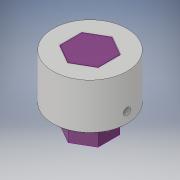
# Autodesk Inventor part: Wheel
Saved by Autodesk Inventor 2019.2 (Build 232265000, 265)
## iProperties
Created: 2019-05-20
Part Number: Wheel
Material: Generic
Document SubType Name: Modeling
Designer: Johansson
Density: 1 g/cm^3
Appearance: Default
Author: Johansson
## iProperties of the stored document Wheel_3DPrint.ipt
Created: 2019-05-23
Part Number: Wheel_3DPrint
Material: Generic
Document SubType Name: Modeling
Designer: Johansson
Density: 1 g/cm^3
Appearance: Default
Author: Johansson
Autodesk Inventor part; units mm, degrees
ref_plane "YZ Plane" through (0, 0, 0) normal (1, 0, 0) x (0, 1, 0)
ref_plane "XZ Plane" through (0, 0, 0) normal (0, 1, 0) x (-1, 0, 0)
ref_plane "XY Plane" through (0, 0, 0) normal (0, 0, 1) x (1, 0, 0)
sketch "Sketch1" plane through (0, 0, 0) normal (0, 1, 0) x (-1, 0, 0)
  circle A0 centre (0, 0) radius 4.1
  line L0 (8.2, 4.7343) -> (8.2, -4.7343)
  line L1 (8.2, -4.7343) -> (0, -9.4685)
  line L2 (0, -9.4685) -> (-8.2, -4.7343)
  line L3 (-8.2, -4.7343) -> (-8.2, 4.7343)
  line L4 (-8.2, 4.7343) -> (0, 9.4685)
  line L5 (0, 9.4685) -> (8.2, 4.7343)
  dimension "d1" = 8.2
  dimension "d5" = 8.2
  constraints: 12 end point, 2 coincident, 1 centre point, 1 vertical, 13 other
  measures "d1" diameter of A0
  measures "d5" distance from line of point (0, 0) L0
extrude "Extrusion1" add sketch "Sketch1" along normal blind 20
sketch "Sketch2" plane through (-8.2, 0, -4.7343) normal (-1, 0, 0) x (0, 0, 1)
  circle A0 centre (4.7343, 5) radius 1.5
  line L0 (9.4685, 0) -> (0, 0) projected
  line L1 (4.7343, -4) -> (4.7343, 24) projected
  point P0 (4.7343, 0)
  dimension "d6" = 3
  dimension "d7" = 5
  constraints: 1 centre point, 1 point on line
  measures "d6" diameter of A0
  measures "d7" distance from line of A0.centre L0
extrude "Extrusion2" cut sketch "Sketch2" against normal through all
ref_plane "Work Plane1" through (0, 10, 0) normal (0, -1, 0) x (1, 0, 0)
mirror "Mirror1" about plane through (0, 10, 0) normal (0, -1, 0) of "Extrusion2"
sketch "Sketch3" plane through (0, 20, 0) normal (0, 1, 0) x (1, 0, 0)
  circle A0 centre (0, 0) radius 4.1 projected
  line L0 (-8.2, 4.7343) -> (-8.2, -4.7343) projected
  line L1 (-8.2, -4.7343) -> (0, -9.4685) projected
  line L2 (0, -9.4685) -> (8.2, -4.7343) projected
  line L3 (8.2, -4.7343) -> (8.2, 4.7343) projected
  line L4 (8.2, 4.7343) -> (0, 9.4685) projected
  line L5 (0, 9.4685) -> (-8.2, 4.7343) projected
  circle A1 centre (0, 0) radius 16
  dimension "d10" = 32
  constraints: 1 centre point, 1 coincident
  measures "d10" diameter of A1
extrude "Extrusion3" add sketch "Sketch3" along normal blind 10 and the other way blind 10 separate body contours A1
thicken "Thicken1" operation add thickness 0.2 both sides no extend neighbours yes toward (0.5, 0, 0.8660254) bodies 2 faces at (2.7333, 23.3333, 7.8905) (2.7333, 16.6667, 7.8905) (-5.4667, 23.3333, 6.3124) (-5.4667, 16.6667, 6.3124) (-8.2, 23.3333, -1.5781) (-8.2, 16.6667, -1.5781) (-2.7333, 26.6667, -7.8905) (-2.7333, 13.3333, -7.8905) (5.4667, 23.3333, -6.3124) (5.4667, 16.6667, -6.3124) (8.2, 23.3333, 1.5781) (8.2, 16.6667, 1.5781)
ref_plane "Work Plane2" through (-16, 20, 0) normal (-1, 0, 0) x (0, -1, 0)
sketch "Sketch4" plane through (-16, 20, 0) normal (-1, 0, 0) x (0, -1, 0)
  circle A0 centre (5, 0) radius 1.5 projected
  point P0 (20, 0)
extrude "Extrusion4" cut sketch "Sketch4" against normal through all bodies 2
sketch "Sketch5" plane through (-8.2, 20, 4.7343) normal (0, 1, 0) x (1, 0, 0)
  point P0 (8.2, 4.7343)
sketch "Sketch6" plane through (0, 20, 0) normal (0, 1, 0) x (1, 0, 0)
  circle A0 centre (0, 0) radius 4.1 projected
  line L0 (-8.2, 4.7343) -> (-8.2, -4.7343) projected
  line L1 (-8.2, -4.7343) -> (0, -9.4685) projected
  line L2 (0, -9.4685) -> (8.2, -4.7343) projected
  line L3 (8.2, -4.7343) -> (8.2, 4.7343) projected
  line L4 (8.2, 4.7343) -> (0, 9.4685) projected
  line L5 (0, 9.4685) -> (-8.2, 4.7343) projected
extrude "Extrusion5" add sketch "Sketch6" along normal up to surface (10 mm away) contours A0 | L5 L4 L3 L2 L1 L0 bodies 1
chamfer "Chamfer1" distance 0.4 angle 45 7 edges at (8.4, 10, 0) (4.2, 10, -7.2746) (-4.2, 10, -7.2746) (-8.4, 10, 0) (-4.2, 10, 7.2746) (4.2, 10, 7.2746) (-16, 10, 0)
equation "\"d5\" = d1"
equation "\"d2\" = W_WheelCenter"
equation "\"d10\" = 4 * D_Shaft_BLDC"
equation "\"d11\" = 0.5 * W_WheelCenter"
equation "\"d12\" = 0.5 * W_WheelCenter"
equation "\"d15\" = T_WheelToShaft"
equation "\"d16\" = T_WheelToShaft"
equation "\"d17\" = 0.666667 * W_WheelCenter"
equation "\"d21\" = 0.666667 * W_WheelCenter"
equation "\"DO_BLDC\" = 63"
equation "\"WO_BLDC\" = 64"
equation "\"D_Shaft_BLDC\" = 8"
equation "\"D_Hole_BLDC\" = 45.5"
equation "\"D_Wheel\" = 235"
equation "\"W_Wall\" = 8"
equation "\"W_WheelCenter\" = 20"
equation "\"T_WheelToShaft\" = 0.2"
body "Solid1"
body "Solid2"
